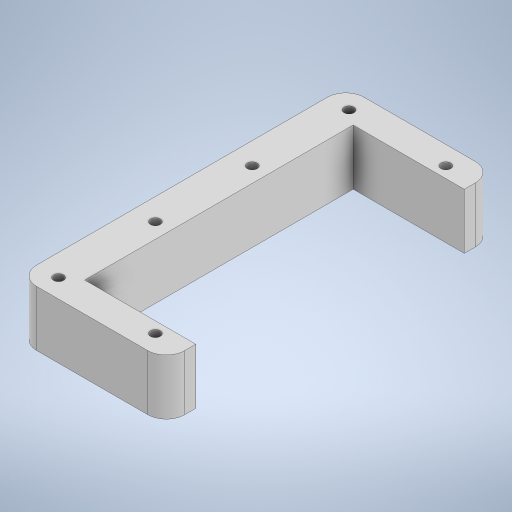
# Autodesk Inventor part: FBH!
Saved by Autodesk Inventor 2024 (Build 280153000, 153)
## iProperties
Created: 2023-08-14
Part Number: FBH!
Material: Generic
Document SubType Name: Modeling
Designer: s137416
Density: 1 g/cm^3
Appearance: Default
Author: s137416
Autodesk Inventor part; units mm, degrees
ref_plane "YZ Plane" through (0, 0, 0) normal (1, 0, 0) x (0, 1, 0)
ref_plane "XZ Plane" through (0, 0, 0) normal (0, 1, 0) x (-1, 0, 0)
ref_plane "XY Plane" through (0, 0, 0) normal (0, 0, 1) x (1, 0, 0)
sketch "Sketch1" plane through (0, 0, 0) normal (0, 1, 0) x (-1, 0, 0)
  line L0 (-50.8, 112.3379) -> (50.8, 112.3379)
  line L1 (50.8, 112.3379) -> (50.8, -112.3378)
  line L2 (50.8, -112.3378) -> (-50.8, -112.3379)
  line L3 (-50.8, -112.3379) -> (-50.8, 112.3379)
  line L4 (-50.8, 112.3379) -> (50.8, -112.3378) construction
  line L5 (50.8, 112.3379) -> (-50.8, -112.3379) construction
  line L6 (-50.8, 92.0813) -> (25.4, 92.0813)
  line L7 (25.4, 92.0813) -> (25.4, -92.0686)
  line L8 (25.4, -92.0686) -> (-50.8, -92.0687)
  line L9 (0, 0) -> (56.1136, 0) construction
  line L10 (76.673, 0) -> (-65.4748, 0)
  line L11 (-31.0246, 99.6379) -> (-31.0246, 0.0063) construction
  line L12 (-31.0246, 0.0063) -> (34.0182, 0.0063) construction
  point P0 (25.4, 0.0063)
  point P1 (-31.0246, -99.6379)
  dimension "d0" = 101.6
  dimension "d56" = 184.15
  dimension "d57" = 76.2
  dimension "d58" = 76.2
  dimension "d60" = 12.7
  dimension "d61" = 12.7
  dimension "d62" = 99.6315
  dimension "d63" = 0
  dimension "d64" = 7.5692
  constraints: 26 end point, 4 perpendicular, 3 horizontal, 3 midpoint, 3 parallel, 3 point on line
  measures "d0" distance of L1.end L2.end
  measures "d56" distance of L6.end L7.end
  measures "d57" distance of L6.start L6.end
  measures "d58" distance of L7.end L8.end
  measures "d60" distance from line of L0 L11.start
  measures "d61" distance from line of L2 point (-31.025, -99.638)
  measures "d62" distance of L11.start L11.end
  measures "d63" distance from line of L12 point (25.4, 0.006)
  measures "d64" distance from line of point (-31.025, -99.638) L8
extrude "Extrusion1" add sketch "Sketch1" along normal blind 38.1 contours L0 L1 L10 L7 L6 L3 | L1 L2 L3 L8 L7 L10
fillet "Fillet1" radius 12.7 4 edges at (50.8, 19.05, 112.3379) (-50.8, 19.05, 112.3379) (-50.8, 19.05, -112.3378) (50.8, 19.05, -112.3379)
sketch "Sketch2" plane through (0, 38.1, 0) normal (0, 1, 0) x (1, 0, 0)
  line L0 (-38.1, -112.3379) -> (38.1, -112.3379) projected
  circle A0 centre (-35.8052, -99.6379) radius 3.3782
  line L1 (-35.8052, -99.6379) -> (-35.8052, 103.5621) construction
  line L2 (-35.8052, -99.6379) -> (40.3948, -99.6379) construction
  line L3 (-35.8052, 103.5621) -> (40.3948, 103.5621) construction
  circle A1 centre (-35.8052, -86.3537) radius 3.3782 construction
  line L4 (-39.1834, -96.2597) -> (-30.0963, -96.2597) construction
  circle A2 centre (-35.8052, -73.0695) radius 3.3782 construction
  circle A3 centre (-35.8052, -59.7853) radius 3.3782 construction
  circle A4 centre (-35.8052, -46.5011) radius 3.3782 construction
  circle A5 centre (-35.8052, -33.2169) radius 3.3782 construction
  circle A6 centre (-35.8052, -19.9327) radius 3.3782 construction
  circle A7 centre (-35.8052, -6.6485) radius 3.3782 construction
  circle A8 centre (-35.8052, 6.6357) radius 3.3782 construction
  circle A9 centre (-35.8052, 19.9199) radius 3.3782 construction
  circle A10 centre (-35.8052, 33.2041) radius 3.3782 construction
  circle A11 centre (-35.8052, 46.4883) radius 3.3782 construction
  circle A12 centre (-35.8052, 59.7725) radius 3.3782 construction
  circle A13 centre (-35.8052, 73.0567) radius 3.3782 construction
  circle A14 centre (-35.8052, 86.3409) radius 3.3782 construction
  circle A15 centre (-35.8052, 99.6251) radius 3.3782 construction
  circle A16 centre (-22.521, -99.6379) radius 3.3782 construction
  circle A17 centre (-9.2368, -99.6379) radius 3.3782 construction
  circle A18 centre (4.0474, -99.6379) radius 3.3782 construction
  circle A19 centre (17.3316, -99.6379) radius 3.3782 construction
  circle A20 centre (30.6158, -99.6379) radius 3.3782 construction
  circle A21 centre (43.9, -99.6379) radius 3.3782 construction
  circle A22 centre (30.6158, 99.6251) radius 3.3782 construction
  circle A23 centre (30.6158, -99.6379) radius 3.3782 construction
  circle A24 centre (-35.8052, 99.6251) radius 3.3782 construction
  circle A25 centre (-35.8052, 33.2041) radius 3.3782 construction
  circle A26 centre (-35.8052, -33.2169) radius 3.3782 construction
  circle A27 centre (-35.8052, -33.2169) radius 3.3782
  circle A28 centre (-35.8052, 33.2041) radius 3.3782
  circle A29 centre (-35.8052, 99.6251) radius 3.3782
  circle A30 centre (30.6158, 99.6251) radius 3.3782
  circle A31 centre (30.6158, -99.6379) radius 3.3782
  point P0 (0, 0)
  point P1 (-35.8052, -23.4379)
  point P2 (-35.8052, 27.3621)
  dimension "d8" = 12.7
  dimension "d9" = 76.2
  dimension "d10" = 127
  dimension "d11" = 203.2
  dimension "d12" = 76.2
  dimension "d13" = 6.7564
  dimension "d22" = 13.2842
  dimension "d25" = 13.2842
  dimension "d30" = 13.2842
  dimension "d33" = 13.2842
  dimension "d38" = 6.7564
  dimension "d39" = 6.7564
  dimension "d40" = 6.7564
  dimension "d41" = 6.7564
  dimension "d42" = 6.7564
  dimension "d43" = 6.7564
  dimension "d44" = 6.7564
  dimension "d45" = 6.7564
  dimension "d46" = 6.7564
  constraints: 32 centre point, 13 coincident, 8 end point, 4 horizontal, 3 equal radius, 2 point on line, 2 vertical, 1 horizontal alignment, 1 tangent, 38 other
  measures "d8" distance from line of L0 point (-35.805, -99.638)
  measures "d9" distance of point (-35.805, -23.438) point (-35.805, -99.638)
  measures "d10" distance of point (-35.805, 27.362) point (-35.805, -99.638)
  measures "d11" distance of point (-35.805, 103.562) point (-35.805, -99.638)
  measures "d12" distance of point (40.395, -99.638) point (-35.805, -99.638)
  measures "d13" diameter of A0
  measures "d22" distance of A1.centre L1.start
  measures "d25" distance of A1.centre A2.centre
  measures "d30" distance of A16.centre L1.start
  measures "d33" distance of A16.centre A17.centre
  measures "d38" diameter of A22
  measures "d39" diameter of A23
  measures "d40" diameter of A24
  measures "d41" diameter of A25
  measures "d42" diameter of A26
  measures "d43" diameter of A28
  measures "d44" diameter of A29
  measures "d45" diameter of A30
  measures "d46" diameter of A31
extrude "Extrusion4" cut sketch "Sketch2" against normal through all
equation "\"d25\" = d22"
equation "\"d30\" = d22"
equation "\"d33\" = d22"
body "Solid1"
